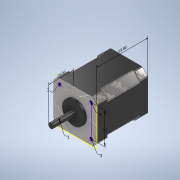
# Autodesk Inventor part: Nema17
Saved by Autodesk Inventor 2020 (Build 240168000, 168)
## iProperties
Created: 2020-02-24
Part Number: Nema17
Material: Типовые
Document SubType Name: Modeling
Designer: andrey
Density: 1 g/cm^3
Appearance: По умолчанию
Author: andrey
Autodesk Inventor part; units mm, degrees
ref_plane "YZ Plane" through (0, 0, 0) normal (1, 0, 0) x (0, 1, 0)
ref_plane "XZ Plane" through (0, 0, 0) normal (0, 1, 0) x (-1, 0, 0)
ref_plane "XY Plane" through (0, 0, 0) normal (0, 0, 1) x (1, 0, 0)
sketch "Эскиз1" plane through (0, 0, 0) normal (0, 0, 1) x (1, 0, 0)
  line L0 (0, 0) -> (42.3, 0)
  line L1 (42.3, 0) -> (42.3, 42.3)
  line L2 (42.3, 42.3) -> (0, 42.3)
  line L3 (0, 42.3) -> (0, 0)
  dimension "d0" = 42.3
  dimension "d1" = 42.3
  constraints: 8 end point, 3 perpendicular, 1 horizontal
  measures "d0" distance of L0.start L0.end
  measures "d1" distance of L0.end L1.end
extrude "Выдавливание1" add sketch "Эскиз1" along normal blind 10
sketch "Эскиз2" plane through (0, 0, 10) normal (0, 0, 1) x (1, 0, 0)
  circle A0 centre (5.65, 5.65) radius 1.5
  circle A1 centre (5.65, 36.65) radius 1.5
  line L0 (0, 0) -> (42.3, 0) projected
  line L1 (42.3, 0) -> (42.3, 42.3) projected
  line L2 (36.65, 5.65) -> (36.65, 36.65)
  circle A2 centre (36.65, 36.65) radius 1.5
  circle A3 centre (36.65, 5.65) radius 1.5
  point P0 (0, 42.3)
  dimension "d6" = 3
  dimension "d7" = 3
  dimension "d12" = 31
  dimension "d13" = 3
  dimension "d14" = 3
  constraints: 4 centre point, 2 coincident, 2 end point, 1 vertical
  measures "d6" diameter of A0
  measures "d7" diameter of A1
  measures "d12" distance of L2.start L2.end
  measures "d13" diameter of A2
  measures "d14" diameter of A3
extrude "Выдавливание2" cut sketch "Эскиз2" against normal blind 4.5
thread "Резьба1" size "M3x0.5" class "6H" standard "ANSI Metric M Profile" full length
thread "Резьба2" size "M3x0.5" class "6H" standard "ANSI Metric M Profile" full length
thread "Резьба3" size "M3x0.5" class "6H" standard "ANSI Metric M Profile" full length
thread "Резьба4" size "M3x0.5" class "6H" standard "ANSI Metric M Profile" full length
sketch "Эскиз3" plane through (0, 0, 10) normal (0, 0, 1) x (1, 0, 0)
  line L0 (0, 42.3) -> (0, 0) projected
  line L1 (0, 42.3) -> (0, 37.8)
  line L2 (0, 0) -> (42.3, 0) projected
  line L3 (0, 0) -> (0, 4.5)
  line L4 (0, 0) -> (4.5, 0)
  line L5 (4.5, 0) -> (0, 4.5)
  line L6 (42.3, 42.3) -> (0, 42.3) projected
  line L7 (0, 42.3) -> (4.5, 42.3)
  line L8 (4.5, 42.3) -> (0, 37.8)
  line L9 (42.3, 42.3) -> (37.8, 42.3)
  line L10 (42.3, 0) -> (42.3, 42.3) projected
  line L11 (42.3, 42.3) -> (42.3, 37.8)
  line L12 (42.3, 37.8) -> (37.8, 42.3)
  line L13 (42.3, 0) -> (37.8, 0)
  line L14 (42.3, 0) -> (42.3, 4.5)
  line L15 (42.3, 4.5) -> (37.8, 0)
  dimension "d27" = 4.5
  dimension "d28" = 4.5
  dimension "d29" = 4.5
  dimension "d30" = 4.5
  dimension "d31" = 4.5
  dimension "d32" = 4.5
  constraints: 24 end point, 9 point on line, 2 perpendicular
  measures "d27" distance of L0.start L1.end
  measures "d28" distance of L0.end L3.end
  measures "d29" distance of L0.end L4.end
  measures "d30" distance of L0.start L7.end
  measures "d31" distance of L6.start L9.end
  measures "d32" distance of L6.start L11.end
extrude "Выдавливание3" cut sketch "Эскиз3" against normal blind 10 contours L6 L8 L0 | L5 L2 L0 | L6 L10 L12 | L15 L10 L2
chamfer "Фаска1" distance 0.5 angle 45 1 edges at (4.5, 42.3, 5)
chamfer "Фаска2" distance 0.5 angle 45 7 edges at (0, 37.8, 5) (37.8, 42.3, 5) (42.3, 37.8, 5) (42.3, 4.5, 5) (37.8, 0, 5) (4.5, 0, 5) (0, 4.5, 5)
sketch "Эскиз5" plane through (0, 0, 0) normal (0, 0, -1) x (-1, 0, 0)
  line L0 (0, 0) -> (-42.3, 0)
  line L1 (-42.3, 0) -> (-42.3, 42.3)
  line L2 (-42.3, 42.3) -> (0, 42.3)
  line L3 (0, 42.3) -> (0, 0)
  line L4 (-42.3, 42.3) -> (-42.3, 35.3)
  line L5 (-42.3, 5) -> (-42.3, 37.3) projected
  line L6 (-42.3, 42.3) -> (-35.3, 42.3)
  line L7 (-37.3, 42.3) -> (-5, 42.3) projected
  line L8 (-35.3, 42.3) -> (-42.3, 35.3)
  line L9 (-42.3, 0) -> (-35.3, 0)
  line L10 (-42.3, 0) -> (-42.3, 7)
  line L11 (-42.3, 7) -> (-35.3, 0)
  line L12 (0, 0) -> (-7, 0)
  line L13 (-5, 0) -> (-37.3, 0) projected
  line L14 (0, 0) -> (0, 7)
  line L15 (0, 7) -> (-7, 0)
  line L16 (0, 42.3) -> (-7, 42.3)
  line L17 (-7, 42.3) -> (0, 35.3)
  line L18 (0, 37.3) -> (0, 5) projected
  dimension "d41" = 42.3
  dimension "d42" = 42.3
  dimension "d43" = 7
  dimension "d44" = 7
  dimension "d45" = 7
  dimension "d46" = 7
  dimension "d47" = 7
  dimension "d48" = 7
  dimension "d49" = 7
  constraints: 30 end point, 9 point on line, 2 parallel, 2 perpendicular, 1 horizontal
  measures "d41" distance of L1.end L2.end
  measures "d42" distance of L0.end L1.end
  measures "d43" distance of L1.end L4.end
  measures "d44" distance of L1.end L6.end
  measures "d45" distance of L0.end L9.end
  measures "d46" distance of L0.end L10.end
  measures "d47" distance of L0.start L12.end
  measures "d48" distance of L0.start L14.end
  measures "d49" distance of L16.start L16.end
extrude "Выдавливание4" add sketch "Эскиз5" along normal blind 32.5 contours L0 L11 L1 L8 L2 L17 L3 L15
chamfer "Фаска3" distance 0.5 angle 45 8 edges at (0, 35.3, -16.25) (7, 42.3, -16.25) (0, 7, -16.25) (7, 0, -16.25) (42.3, 35.3, -16.25) (35.3, 42.3, -16.25) (42.3, 7, -16.25) (35.3, 0, -16.25)
sketch "Эскиз10" plane through (0, 0, -32.5) normal (0, 0, -1) x (-1, 0, 0)
  line L0 (0, 0) -> (-42.3, 0)
  line L1 (-42.3, 0) -> (-42.3, 42.3)
  line L2 (-42.3, 42.3) -> (0, 42.3)
  line L3 (0, 42.3) -> (0, 0)
  line L4 (-42.3, 42.3) -> (-36.65, 42.3)
  line L5 (-42.3, 42.3) -> (-42.3, 36.65)
  line L6 (-42.3, 36.65) -> (-36.65, 42.3)
  line L7 (0, 42.3) -> (-5.65, 42.3)
  line L8 (0, 42.3) -> (0, 36.65)
  line L9 (0, 36.65) -> (-5.65, 42.3)
  line L10 (-37.3, 42.3) -> (-5, 42.3) projected
  line L11 (0, 0) -> (-5.65, 0)
  line L12 (0, 0) -> (0, 5.65)
  line L13 (0, 7.5) -> (0, 5) projected
  line L14 (0, 5.65) -> (-5.65, 0)
  line L15 (-42.3, 0) -> (-42.3, 5.65)
  line L16 (-42.3, 0) -> (-36.65, 0)
  line L17 (-35.6536, 0.3536) -> (-41.9464, 6.6464) projected
  line L18 (-36.65, 0) -> (-42.3, 5.65)
  dimension "d57" = 42.3
  dimension "d58" = 42.3
  dimension "d59" = 5.65
  dimension "d60" = 5.65
  dimension "d61" = 5.65
  dimension "d62" = 5.65
  dimension "d63" = 5.65
  dimension "d64" = 5.65
  dimension "d65" = 5.65
  dimension "d66" = 5.65
  constraints: 32 end point, 9 point on line, 2 parallel, 1 horizontal, 1 perpendicular
  measures "d57" distance of L1.end L2.end
  measures "d58" distance of L0.end L1.end
  measures "d59" distance of L1.end L4.end
  measures "d60" distance of L1.end L5.end
  measures "d61" distance of L2.end L7.end
  measures "d62" distance of L2.end L8.end
  measures "d63" distance of L0.start L11.end
  measures "d64" distance of L0.start L12.end
  measures "d65" distance of L0.end L15.end
  measures "d66" distance of L0.end L16.end
extrude "Выдавливание5" add sketch "Эскиз10" along normal blind 7.5 contours L0 L18 L1 L6 L2 L9 L3 L14
chamfer "Фаска4" distance 0.5 angle 45 8 edges at (0, 36.65, -36.25) (5.65, 42.3, -36.25) (0, 5.65, -36.25) (5.65, 0, -36.25) (36.65, 0, -36.25) (42.3, 5.65, -36.25) (36.65, 42.3, -36.25) (42.3, 36.65, -36.25)
sketch "Эскиз11" plane through (0, 0, -40) normal (0, 0, -1) x (-1, 0, 0)
  circle A0 centre (-5.65, 5.65) radius 1.5 projected
  circle A1 centre (-5.65, 5.65) radius 1.5
  circle A2 centre (-36.65, 5.65) radius 1.5 projected
  circle A3 centre (-36.65, 5.65) radius 1.5
  circle A4 centre (-36.65, 36.65) radius 1.5 projected
  circle A5 centre (-36.65, 36.65) radius 1.5
  circle A6 centre (-5.65, 36.65) radius 1.5 projected
  circle A7 centre (-5.65, 36.65) radius 1.5
  point P0 (0, 0)
  constraints: 4 centre point, 4 coincident
extrude "Выдавливание6" cut sketch "Эскиз11" against normal blind 4
thread "Резьба5" size "M3x0.5" class "6H" standard "ANSI Metric M Profile" full length
thread "Резьба6" size "M3x0.5" class "6H" standard "ANSI Metric M Profile" full length
thread "Резьба7" size "M3x0.5" class "6H" standard "ANSI Metric M Profile" full length
thread "Резьба8" size "M3x0.5" class "6H" standard "ANSI Metric M Profile" full length
sketch "Эскиз12" plane through (0, 0, 10) normal (0, 0, 1) x (1, 0, 0)
  line L0 (0, 0) -> (42.3, 0)
  line L1 (42.3, 0) -> (42.3, 42.3)
  line L2 (42.3, 42.3) -> (0, 42.3)
  line L3 (0, 42.3) -> (0, 0)
  line L4 (0, 42.3) -> (42.3, 0)
  line L5 (0, 0) -> (42.3, 42.3)
  circle A0 centre (21.15, 21.15) radius 11
  dimension "d82" = 42.3
  dimension "d83" = 42.3
  dimension "d84" = 22
  constraints: 12 end point, 2 parallel, 1 centre point, 1 horizontal, 1 midpoint, 1 perpendicular
  measures "d82" distance of L2.end L1.end
  measures "d83" distance of L1.end L0.end
  measures "d84" diameter of A0
extrude "Выдавливание7" add sketch "Эскиз12" along normal blind 2 contours A0 L4 L5 | L5 L4 A0 | L4 L5 A0 | A0 L5 L4
sketch "Эскиз13" plane through (21.15, 21.15, 12) normal (0, 0, 1) x (1, 0, 0)
  circle A0 centre (0, 0) radius 2.5
  point P0 (-21.15, -21.15)
  dimension "d87" = 5
  constraints: 1 centre point
  measures "d87" diameter of A0
extrude "Выдавливание8" add sketch "Эскиз13" along normal blind 22
